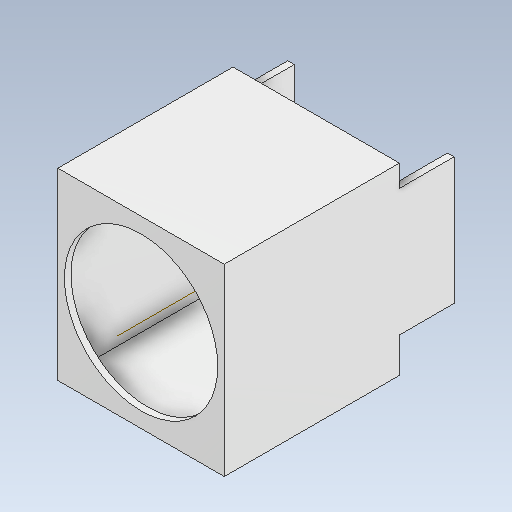
# Autodesk Inventor part: EStop Mount
Saved by Autodesk Inventor 2020 (Build 240168000, 168)
## iProperties
Created: 2020-02-04
Part Number: EStop Mount
Material: PBT Plastic
Document SubType Name: Modeling
Designer: GJCla
Density: 1.31 g/cm^3
Appearance: Smooth - White
Author: GJCla
Autodesk Inventor part; units mm, degrees
ref_plane "YZ Plane" through (0, 0, 0) normal (1, 0, 0) x (0, 1, 0)
ref_plane "XZ Plane" through (0, 0, 0) normal (0, 1, 0) x (-1, 0, 0)
ref_plane "XY Plane" through (0, 0, 0) normal (0, 0, 1) x (1, 0, 0)
sketch "Sketch1" plane through (0, 0, 0) normal (0, 0, 1) x (1, 0, 0)
  line L0 (24.13, -26.67) -> (-24.13, -26.67)
  line L1 (-24.13, -26.67) -> (-24.13, 26.67)
  line L2 (-24.13, 26.67) -> (24.13, 26.67)
  line L3 (24.13, 26.67) -> (24.13, -26.67)
  line L4 (0, 37.338) -> (0, -37.338) projected
  line L5 (-33.782, 0) -> (33.782, 0) projected
  dimension "d0" = 53.34
  dimension "d1" = 48.26
  constraints: 8 end point, 2 parallel, 1 horizontal, 1 perpendicular, 2 other
  measures "d0" distance of L0.end L1.end
  measures "d1" distance between parallel lines of L3 L1
extrude "Extrusion1" add sketch "Sketch1" against normal blind 66.675
shell "Shell1" thickness 1.905 removed faces 1 at (-8.0433, 8.89, -66.675)
sketch "Sketch2" plane through (0, 0, 0) normal (0, 0, 1) x (1, 0, 0)
  point P0 (0, 0)
  point P1 (0, 0)
  constraints: 1 coincident
hole "Hole1" at (0, 0, 0) direction (0, 0, -1) diameter 44.45 end through all
sketch "Sketch3" plane through (24.13, -26.67, 0) normal (1, 0, 0) x (0, 0, -1)
  line L0 (0, 0) -> (66.675, 0) projected
  line L1 (50.8, 0) -> (50.8, 10.16)
  line L2 (50.8, 10.16) -> (66.675, 10.16)
  line L3 (66.675, 1.905) -> (66.675, 51.435) projected
  line L4 (0, 53.34) -> (66.675, 53.34) projected
  line L5 (50.8, 53.34) -> (50.8, 46.99)
  line L6 (50.8, 46.99) -> (66.675, 46.99)
  line L7 (66.675, 53.34) -> (66.675, 0) projected
  point P0 (0, 26.67)
  dimension "d12" = 10.16
  dimension "d13" = 6.35
  dimension "d14" = 15.875
  constraints: 8 end point, 6 point on line, 2 perpendicular, 1 vertical
  measures "d12" distance of L1.start L1.end
  measures "d13" distance of L5.start L5.end
  measures "d14" distance of L5.end L6.end
extrude "Extrusion2" cut sketch "Sketch3" against normal up to next
body "Solid1"
